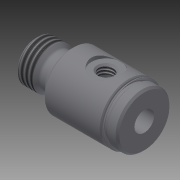
# Autodesk Inventor part: D-26368----0.5_rod_guide_cyl
Saved by Autodesk Inventor 2014 (Build 180170000, 170)
## iProperties
Created: 2014-01-19
Part Number: D-26368----0.5_rod_guide_cyl
Material: Generic
Catalog Web Link: www.cadenas.de
Description: Rod Guide Cyl-Original Line Cyl
Vendor: BIMBA
Document SubType Name: Standard Catalog Part
Designer: Michael
Manufacturer: BIMBA
Density: 1 g/cm^3
Appearance: RGB(211.00000262260440,211.00000262260440,211.00000262260440)
Category: PARTsolutions
Company: BIMBA
Title: D-26368----0.5_rod_guide_cyl
Author: Cadenas PARTsolutions
Comments: Original Line Cyl
PSOL_IDENT_0: {$CADENAS_DATA\23d-libs\bimba\bimba\bimba_imperial\bimba_full_line\original_line_cylinders\three_pos
PSOL_IDENT_1: ition_cylinders\rod_guide_cyl.prj},219 {VTYP=3D},{NB=D-26368----0.5_rod_guide_cyl},{LINA=D-26368----
PSOL_IDENT_2: 0.5_rod_guide_cyl},{NN=Rod Guide Cyl},{DATE=19.03.2013 10:15:23},{GEOMDATE=19.03.2013 11:15:00},{VER
PSOL_IDENT_3: SION=},{LINEID=30},{LINESUBID=-1},{WBVAR=NR,NT,RODTRANS}  {NB=D-26368----0.5_rod_guide_cyl},{LINA=D-
PSOL_IDENT_4: 26368----0.5_rod_guide_cyl},{KT=DUMMY},{PN=D-26368},{BORE=0.56250000},{BOREPN=02},{MNT=},{ACTING=R},
PSOL_IDENT_5: {NR=},{NRALG= '' , 'Without Non-rotating Rod' , 'NR' , 'With Non-rotating Rod' },{K=},{NT=},{A1=1.15
PSOL_IDENT_6: 60},{A1N=1.0310},{A1P=1.1560},{A1B=0.0000},{A2=0.3750},{A2N=0.3750},{A2P=0.3750},{A3=0.6250},{A3N=0.
PSOL_IDENT_7: 1250},{A3P=0.6250},{A4=0.1570},{A4N=0.5310},{A4P=0.1570},{A5=0.0250},{A6=0.0000},{A6N=0.2810},{A6P=0
PSOL_IDENT_8: .0000},{A7=0.5000},{A7N=0.6560},{A7P=0.5000},{A8=0.0200},{A8N=0.0200},{A8NR=0.0200},{D1=0.6150},{D1N=
PSOL_IDENT_9: 0.6150},{D1P=0.6150},{D1B=0.0000},{D2=0.5730},{D3=0.0000},{D3N=0.4000},{D3P=0.0000},{D4=0.3440},{D4N=
PSOL_IDENT_10: 0.2220},{D4P=0.3440},{D4NR=0.3440},{HEXN=0.1900},{D5=0.1900},{D5N=0.1900},{D5NR=0.1900},{C1=0.030},{
PSOL_IDENT_11: C2=0.0200},{C2N=0.0300},{C2P=0.0200},{C3=0.0100},{C3N=0.0100},{C3P=0.0100},{C4=0.0300},{C4N=0.0300},
PSOL_IDENT_12: {C4P=0.0300},{NDM=0.4375},{NDMN=0.4375},{NDMP=0.4375},{TAB=UNF},{D6=0.4355},{D6N=0.4355},{D6P=0.4355
PSOL_IDENT_13: },{A9=0.0600},{A9N=0.0600},{A9P=0.0600},{D7=0.3600},{D7N=0.3600},{D7P=0.3600},{A10=0.0775},{A10N=0.0
PSOL_IDENT_14: 775},{A10P=0.0775},{R1=0.0315},{R1N=0.0315},{R1P=0.0315},{D8=0.0000},{D9=0.0000},{D10=0.0000},{A11=0
PSOL_IDENT_15: .0000},{A12=0.0000},{A13=0.0000},{A14=0.4060},{A14N=0.4060},{A14B=0.0000},{D11=0.0000},{D11N=0.0000}
PSOL_IDENT_16: ,{NDM2=0.1900},{NDM2N=0.1900},{NDM2DP=0.0000},{THREAD=0},{HEX=0.1900},{S1=0.0000},{B1=0.0000},{B2=0.
PSOL_IDENT_17: 0000},{B22=0.0000},{DB=0.0000},{B3=0.0000},{B4=0.0000},{X1=0.0000},{X2=0.0000},{NDM3=0.0000},{NDM4=0
PSOL_IDENT_18: .0000},{NDM4DP=0.0000},{DD=0.0000},{CB=0.0000},{CBDP=0.0000},{PORT=1},{XT=0.0000},{XT1=0.0000},{XT2=
PSOL_IDENT_19: 0.0000},{NDMH=0.0000},{OD=0.6150},{ID=0.5730},{G=0.0000},{RP=0.15385700},{D=0.27000000},{DD1=0.21600
PSOL_IDENT_20: 000},{CH1=0.10700000},{RODTRANS=0.50000}
CNS_NN: Rod Guide Cyl
CNS_NT: Standard
CNS_NB: D-26368----0.5_rod_guide_cyl
CNS_NBSYN: $PN.-$NR.-$K.-$NT.-$RODTRANS._rod_guide_cyl
CNS_LINA: D-26368----0.5_rod_guide_cyl
CNS_PN: D-26368
CNS_BORE: 9/16
CNS_BOREPN: 02
CNS_ACTING: R
CNS_NR: Without Non-rotating Rod
CNS_NRALG: '' , 'Without Non-rotating Rod' , 'NR' , 'With Non-rotating Rod'
CNS_A1: 1.1560
CNS_A1N: 1.0310
CNS_A1P: 1.1560
CNS_A1B: 0.0000
CNS_A2: 0.3750
CNS_A2N: 0.3750
CNS_A2P: 0.3750
CNS_A3: 0.6250
CNS_A3N: 0.1250
CNS_A3P: 0.6250
CNS_A4: 0.1570
CNS_A4N: 0.5310
CNS_A4P: 0.1570
CNS_A5: 0.0250
CNS_A6: 0.0000
CNS_A6N: 0.2810
CNS_A6P: 0.0000
CNS_A7: 0.5000
CNS_A7N: 0.6560
CNS_A7P: 0.5000
CNS_A8: 0.0200
CNS_A8N: 0.0200
CNS_A8NR: 0.0200
CNS_D1: 0.6150
CNS_D1N: 0.6150
CNS_D1P: 0.6150
CNS_D1B: 0.0000
CNS_D2: 0.5730
CNS_D3: 0.0000
CNS_D3N: 0.4000
CNS_D3P: 0.0000
CNS_D4: 0.3440
CNS_D4N: 0.2220
CNS_D4P: 0.3440
CNS_D4NR: 0.3440
CNS_HEXN: 0.1900
CNS_D5: 0.1900
CNS_D5N: 0.1900
CNS_D5NR: 0.1900
CNS_C1: 0.030
CNS_C2: 0.0200
CNS_C2N: 0.0300
CNS_C2P: 0.0200
CNS_C3: 0.0100
CNS_C3N: 0.0100
CNS_C3P: 0.0100
CNS_C4: 0.0300
CNS_C4N: 0.0300
CNS_C4P: 0.0300
CNS_NDM: 0.4375
CNS_NDMN: 0.4375
CNS_NDMP: 0.4375
CNS_TAB: UNF
CNS_D6: 0.4355
CNS_D6N: 0.4355
CNS_D6P: 0.4355
CNS_A9: 0.0600
CNS_A9N: 0.0600
CNS_A9P: 0.0600
CNS_D7: 0.3600
CNS_D7N: 0.3600
CNS_D7P: 0.3600
CNS_A10: 0.0775
CNS_A10N: 0.0775
CNS_A10P: 0.0775
CNS_R1: 0.0315
CNS_R1N: 0.0315
CNS_R1P: 0.0315
CNS_D8: 0.0000
CNS_D9: 0.0000
CNS_D10: 0.0000
CNS_A11: 0.0000
CNS_A12: 0.0000
CNS_A13: 0.0000
CNS_A14: 0.4060
CNS_A14N: 0.4060
CNS_A14B: 0.0000
CNS_D11: 0.0000
CNS_D11N: 0.0000
CNS_NDM2: 0.1900
CNS_NDM2N: 0.1900
CNS_NDM2DP: 0.0000
CNS_THREAD: 0
CNS_HEX: 0.1900
CNS_S1: 0.0000
CNS_B1: 0.0000
CNS_B2: 0.0000
CNS_B22: 0.0000
CNS_DB: 0.0000
CNS_B3: 0.0000
CNS_B4: 0.0000
CNS_X1: 0.0000
CNS_X2: 0.0000
CNS_NDM3: 0.0000
CNS_NDM4: 0.0000
CNS_NDM4DP: 0.0000
CNS_DD: 0.0000
CNS_CB: 0.0000
CNS_CBDP: 0.0000
CNS_PORT: 1
CNS_XT: 0.0000
CNS_XT1: 0.0000
CNS_XT2: 0.0000
CNS_NDMH: 0.0000
CNS_OD: 0.6150
CNS_ID: 0.5730
CNS_G: 0.0000
CNS_RP: 0.15385700
CNS_D: 0.27000000
CNS_DD1: 0.21600000
CNS_CH1: 0.10700000
CNS_RODTRANS: 0.50000
SUPPLIER: BIMBA
ARTICLENO: D-26368----0.5_rod_guide_cyl
BOMINFO: D-26368----0.5_rod_guide_cyl
CREATOR: CADENAS GmbH
Autodesk Inventor part; units mm, degrees
ref_plane "YZ Plane" through (0, 0, 0) normal (1, 0, 0) x (0, 1, 0)
ref_plane "XZ Plane" through (0, 0, 0) normal (0, 1, 0) x (-1, 0, 0)
ref_plane "XY Plane" through (0, 0, 0) normal (0, 0, 1) x (1, 0, 0)
sketch "Sketch_2" plane through (0, 0, 0) normal (0, 0, 1) x (1, 0, 0)
  line L0 (9.525, 0) -> (0, 0)
  line L1 (0, 0) -> (0, 4.8006)
  line L2 (0, 4.8006) -> (0.7556, 5.5563)
  line L3 (0.7556, 5.5563) -> (4.7111, 5.5563)
  line L4 (4.7111, 5.5563) -> (5.4689, 4.8042)
  arc A0 (5.4689, 4.8042) -> (6.0325, 4.572) centre (6.0325, 5.3721) ccw
  line L5 (6.0325, 4.572) -> (7.2009, 4.572)
  arc A1 (7.2009, 4.572) -> (8.001, 5.3721) centre (7.2009, 5.3721) ccw
  line L6 (8.001, 5.3721) -> (8.001, 5.5309)
  line L7 (8.001, 5.5309) -> (9.525, 5.5309)
  line L8 (9.525, 5.5309) -> (9.525, 0)
  line L9 (9.525, 0) -> (0, 0)
  constraints: 20 end point, 4 point on circle, 2 centre point
revolve "Revolution1" add sketch "Sketch_2" angle 360 about axis through (9.525, 0, 0) along (1, 0, 0)
thread "Thread1" size "7/16-20 UNF" class "2A" standard "ANSI Unified Screw Threads" full length
sketch "Sketch_3" plane through (0, 0, 0) normal (0, 0, 1) x (1, 0, 0)
  line L0 (29.3624, 0) -> (9.525, 0)
  line L1 (9.525, 0) -> (9.525, 7.0485)
  line L2 (9.525, 7.0485) -> (10.287, 7.8105)
  line L3 (10.287, 7.8105) -> (25.1206, 7.8105)
  line L4 (25.1206, 7.8105) -> (25.3746, 7.5565)
  line L5 (25.3746, 7.5565) -> (25.3746, 6.6421)
  line L6 (25.3746, 6.6421) -> (26.0096, 6.6421)
  line L7 (26.0096, 6.6421) -> (26.6446, 7.2771)
  line L8 (26.6446, 7.2771) -> (28.8544, 7.2771)
  line L9 (28.8544, 7.2771) -> (29.3624, 6.7691)
  line L10 (29.3624, 6.7691) -> (29.3624, 0)
  line L11 (29.3624, 0) -> (9.525, 0)
  constraints: 24 end point
revolve "Revolution2" add sketch "Sketch_3" angle 360 about axis through (29.3624, 0, 0) along (1, 0, 0)
sketch "Sketch3" plane through (0, 0, 0) normal (-1, 0, 0) x (0, 0, 1)
  point P0 (0, 0)
hole "Hole1" at (0, 0, 0) direction (1, 0, 0) diameter 5.334 depth 29.3624 countersink diameter 6.35 countersink angle 90
sketch "Sketch_13" plane through (0, 0, 0) normal (0, 0, 1) x (1, 0, 0)
  line L0 (19.05, -1.016) -> (19.05, 7.8105)
  line L1 (19.05, 7.8105) -> (23.0124, 7.8105)
  line L2 (23.0124, 7.8105) -> (23.0124, 6.7945)
  line L3 (23.0124, 6.7945) -> (21.463, 6.7945)
  line L4 (21.463, 6.7945) -> (21.0337, 6.3652)
  line L5 (21.0337, 6.3652) -> (21.0337, -1.016)
  line L6 (21.0337, -1.016) -> (19.05, -1.016)
  line L7 (19.05, -1.016) -> (19.05, 7.8105)
  constraints: 16 end point
revolve "Revolution3" cut sketch "Sketch_13" angle 360 about axis through (19.05, -1.016, 0) along (0, -1, 0)
thread "Thread2" size "10-32 UNF" class "2B" standard "ANSI Unified Screw Threads" length 2.4257 offset 2.5862
sketch "Sketch_47" plane through (0, 0, 0) normal (0, 0, 1) x (1, 0, 0)
  line L0 (29.3624, 0) -> (-29.3624, 0)
  line L1 (24.8242, 6.6421) -> (25.1116, 6.6421)
  line L2 (25.1116, 6.6421) -> (26.1958, 7.7263)
  line L3 (26.1958, 7.7263) -> (26.1958, 7.8105)
  line L4 (26.1958, 7.8105) -> (25.9926, 7.8105)
  line L5 (25.9926, 7.8105) -> (24.8242, 6.6421)
  constraints: 12 end point
revolve "Revolution4" add sketch "Sketch_47" angle 360 about axis through (29.3624, 0, 0) along (1, 0, 0)
ref_plane "c2_XY" through (19.05, 0, 0) normal (0, 0, 1) x (1, 0, 0)
ref_plane "c2_YZ" through (19.05, 0, 0) normal (1, 0, 0) x (0, 1, 0)
ref_plane "c2_ZX" through (19.05, 0, 0) normal (0, 1, 0) x (0, 0, 1)
ref_plane "e2_XY" through (9.525, 0, 0) normal (0, 0, 1) x (1, 0, 0)
ref_plane "e2_YZ" through (9.525, 0, 0) normal (1, 0, 0) x (0, 1, 0)
ref_plane "e2_ZX" through (9.525, 0, 0) normal (0, 1, 0) x (0, 0, 1)
ref_plane "f1_XY" through (8.001, 0, 0) normal (0, 0, 1) x (1, 0, 0)
ref_plane "f1_YZ" through (8.001, 0, 0) normal (1, 0, 0) x (0, 1, 0)
ref_plane "f1_ZX" through (8.001, 0, 0) normal (0, 1, 0) x (0, 0, 1)
ref_plane "f2_XY" through (9.525, 0, 0) normal (0, 0, 1) x (1, 0, 0)
ref_plane "f2_YZ" through (9.525, 0, 0) normal (1, 0, 0) x (0, 1, 0)
ref_plane "f2_ZX" through (9.525, 0, 0) normal (0, 1, 0) x (0, 0, 1)
ref_plane "i1_XY" through (0, 0, -5.5563) normal (0, 1, 0) x (1, 0, 0)
ref_plane "i1_YZ" through (0, 0, -5.5563) normal (1, 0, 0) x (0, 0, -1)
ref_plane "i1_ZX" through (0, 0, -5.5563) normal (0, 0, -1) x (0, 1, 0)
ref_plane "i2_XY" through (0, 0, 5.5563) normal (0, 1, 0) x (1, 0, 0)
ref_plane "i2_YZ" through (0, 0, 5.5563) normal (1, 0, 0) x (0, 0, -1)
ref_plane "i2_ZX" through (0, 0, 5.5563) normal (0, 0, -1) x (0, 1, 0)
ref_plane "l1_XY" through (9.525, 0, -5.5309) normal (0, 1, 0) x (1, 0, 0)
ref_plane "l1_YZ" through (9.525, 0, -5.5309) normal (1, 0, 0) x (0, 0, -1)
ref_plane "l1_ZX" through (9.525, 0, -5.5309) normal (0, 0, -1) x (0, 1, 0)
ref_plane "l2_XY" through (9.525, 0, 5.5309) normal (0, 1, 0) x (1, 0, 0)
ref_plane "l2_YZ" through (9.525, 0, 5.5309) normal (1, 0, 0) x (0, 0, -1)
ref_plane "l2_ZX" through (9.525, 0, 5.5309) normal (0, 0, -1) x (0, 1, 0)
ref_plane "rod_guide_XY" through (0, 0, 0) normal (1, 0, 0) x (0, 0, -1)
ref_plane "rod_guide_YZ" through (0, 0, 0) normal (0, 0, -1) x (0, 1, 0)
ref_plane "rod_guide_ZX" through (0, 0, 0) normal (0, 1, 0) x (1, 0, 0)
ref_plane "to_mounting_bracket_XY" through (9.525, 0, 0) normal (1, 0, 0) x (0, 0, -1)
ref_plane "to_mounting_bracket_YZ" through (9.525, 0, 0) normal (0, 0, -1) x (0, 1, 0)
ref_plane "to_mounting_bracket_ZX" through (9.525, 0, 0) normal (0, 1, 0) x (1, 0, 0)
ref_plane "to_rod_XY" through (-12.7, 0, 0) normal (1, 0, 0) x (0, 0, -1)
ref_plane "to_rod_YZ" through (-12.7, 0, 0) normal (0, 0, -1) x (0, 1, 0)
ref_plane "to_rod_ZX" through (-12.7, 0, 0) normal (0, 1, 0) x (1, 0, 0)
ref_plane "to_tube_XY" through (26.6446, 0, 0) normal (1, 0, 0) x (0, 0, -1)
ref_plane "to_tube_YZ" through (26.6446, 0, 0) normal (0, 0, -1) x (0, 1, 0)
ref_plane "to_tube_ZX" through (26.6446, 0, 0) normal (0, 1, 0) x (1, 0, 0)
body "Solid1"
